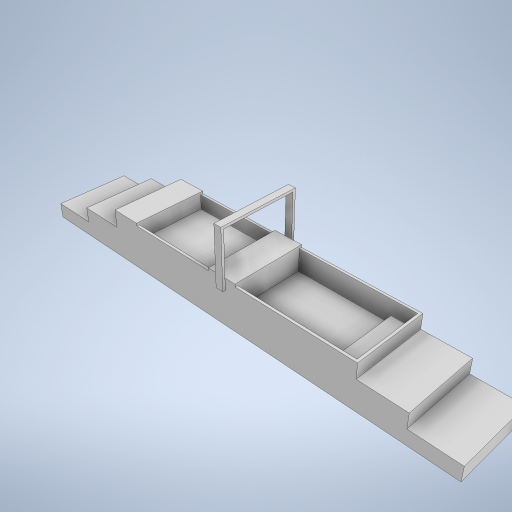
# Autodesk Inventor part: platform
Saved by Autodesk Inventor 2023 (Build 270158000, 158)
## iProperties
Created: 2022-10-30
Part Number: platform
Material: Generic
Document SubType Name: Modeling
Designer: omrfrkmll
Density: 1 g/cm^3
Appearance: Default
Author: omrfrkmll
Autodesk Inventor part; units mm, degrees
ref_plane "YZ Plane" through (0, 0, 0) normal (1, 0, 0) x (0, 1, 0)
ref_plane "XZ Plane" through (0, 0, 0) normal (0, 1, 0) x (-1, 0, 0)
ref_plane "XY Plane" through (0, 0, 0) normal (0, 0, 1) x (1, 0, 0)
sketch "Sketch1" plane through (0, 0, 0) normal (0, 0, 1) x (1, 0, 0)
  line L0 (0, 0) -> (0, 100)
  line L1 (0, 100) -> (300, 100)
  line L2 (300, 100) -> (300, 200)
  line L3 (300, 200) -> (600, 200)
  line L4 (600, 200) -> (600, 300)
  line L5 (2400, 300) -> (2400, 200)
  line L6 (2400, 200) -> (2700, 200)
  line L7 (2700, 200) -> (2700, 100)
  line L8 (2700, 100) -> (3000, 100)
  line L9 (3000, 100) -> (3000, 0)
  line L10 (3000, 0) -> (0, 0)
  line L11 (1600, 300) -> (1600, 318)
  line L12 (1600, 318) -> (1400, 318)
  line L13 (1400, 318) -> (1400, 300)
  line L14 (800, 300) -> (1400, 300)
  line L15 (1600, 300) -> (2400, 300)
  line L16 (800, 300) -> (800, 318)
  line L17 (800, 318) -> (600, 318)
  line L18 (600, 318) -> (600, 300)
  dimension "d0" = 100
  dimension "d1" = 100
  dimension "d2" = 300
  dimension "d6" = 300
  dimension "d7" = 300
  dimension "d10" = 18
  dimension "d11" = 18
  dimension "d12" = 100
  dimension "d13" = 800
  dimension "d15" = 300
  dimension "d16" = 800
  dimension "d17" = 200
  dimension "d44" = 200
  constraints: 38 end point, 14 perpendicular, 4 point on line, 2 vertical, 1 parallel
  measures "d0" distance between parallel lines of L10 L1
  measures "d1" distance between parallel lines of L1 L3
  measures "d2" distance between parallel lines of L0 L2
  measures "d6" distance between parallel lines of L5 L7
  measures "d7" distance between parallel lines of L7 L9
  measures "d10" distance between parallel lines of L12 L14
  measures "d11" distance of L11.start L11.end
  measures "d12" distance between parallel lines of L6 L15
  measures "d13" distance between parallel lines of L11 L5
  measures "d15" distance between parallel lines of L4 L2
  measures "d16" distance between parallel lines of L13 L4
  measures "d17" distance between parallel lines of L13 L11
  measures "d44" distance between parallel lines of L16 L18
extrude "Extrusion1" add sketch "Sketch1" along normal blind 500
sketch "Sketch2" plane through (1600, 300, 0) normal (0, 1, 0) x (1, 0, 0)
  line L0 (0, -18) -> (782, -18)
  line L1 (782, -18) -> (782, -482)
  line L2 (782, -482) -> (0, -482)
  line L3 (0, -482) -> (0, -18)
  line L4 (800, -500) -> (0, -500) projected
  line L5 (800, 0) -> (0, 0) projected
  line L6 (0, 0) -> (0, -500) projected
  line L7 (800, 0) -> (800, -500) projected
  point P0 (-1600, 0)
  point P1 (800, -250)
  dimension "d18" = 18
  dimension "d19" = 18
  dimension "d21" = 0
  dimension "d22" = 18
  constraints: 8 end point, 2 parallel, 1 horizontal, 1 midpoint, 1 perpendicular
  measures "d18" distance between parallel lines of L4 L2
  measures "d19" distance between parallel lines of L5 L0
  measures "d21" distance between parallel lines of L6 L3
  measures "d22" distance from line of point (800, -250) L1
extrude "Extrusion2" cut sketch "Sketch2" against normal blind 100 contours L0 L1 L2 L3
sketch "Sketch3" plane through (1600, 200, 0) normal (0, 1, 0) x (1, 0, 0)
  line L0 (0, 0) -> (0, -500) projected
  line L1 (0, -18) -> (632, -18)
  line L2 (632, -18) -> (632, -482)
  line L3 (632, -482) -> (0, -482)
  line L4 (0, -482) -> (0, -18)
  line L5 (0, -18) -> (782, -18) projected
  line L6 (782, -482) -> (0, -482) projected
  line L7 (782, -18) -> (782, -482) projected
  point P0 (-1600, 0)
  point P1 (0, -482)
  dimension "d25" = 0
  dimension "d26" = 0
  dimension "d27" = 150
  constraints: 8 end point, 2 parallel, 1 horizontal, 1 perpendicular, 1 point on line
  measures "d25" distance between parallel lines of L5 L1
  measures "d26" distance between parallel lines of L6 L3
  measures "d27" distance between parallel lines of L7 L2
extrude "Extrusion3" cut sketch "Sketch3" against normal blind 50 contours L1 L2 L3 L0
sketch "Sketch4" plane through (600, 300, 0) normal (0, 1, 0) x (1, 0, 0)
  line L0 (800, 0) -> (800, -500) projected
  line L1 (800, -18) -> (200, -18)
  line L2 (200, -18) -> (200, -482)
  line L3 (200, -482) -> (800, -482)
  line L4 (800, -482) -> (800, -18)
  line L5 (800, 0) -> (200, 0) projected
  line L6 (800, -500) -> (200, -500) projected
  line L7 (0, 0) -> (0, -500) projected
  point P0 (-600, 0)
  point P1 (800, -482)
  dimension "d30" = 18
  dimension "d31" = 18
  dimension "d32" = 200
  constraints: 8 end point, 2 parallel, 1 horizontal, 1 perpendicular, 1 point on line
  measures "d30" distance between parallel lines of L5 L1
  measures "d31" distance between parallel lines of L6 L3
  measures "d32" distance between parallel lines of L7 L2
extrude "Extrusion4" cut sketch "Sketch4" against normal blind 100
ref_plane "Work Plane1" through (1400, 238, 0) normal (0, 1, 0) x (1, 0, 0)
sketch "Sketch5" plane through (1400, 238, 0) normal (0, 1, 0) x (1, 0, 0)
  line L0 (200, 0) -> (0, 0) projected
  line L1 (125, 0) -> (75, 0)
  line L2 (75, 0) -> (75, 18)
  line L3 (75, 18) -> (125, 18)
  line L4 (125, 18) -> (125, 0)
  line L5 (0, 0) -> (0, -500) projected
  line L6 (0, -250) -> (1064.6178, -250)
  line L7 (200, -500) -> (0, -500) projected
  line L8 (100, -500) -> (100, 124.9847)
  line L9 (125, -500) -> (75, -500)
  line L10 (75, -500) -> (75, -518)
  line L11 (75, -518) -> (125, -518)
  line L12 (125, -518) -> (125, -500)
  point P0 (-1400, 0)
  dimension "d36" = 50
  dimension "d37" = 18
  constraints: 20 end point, 4 symmetric about line, 2 horizontal, 2 midpoint, 2 parallel, 1 perpendicular, 1 point on line, 1 vertical, 1 other
  measures "d36" distance between parallel lines of L4 L2
  measures "d37" distance between parallel lines of L0 L3
extrude "Extrusion5" add sketch "Sketch5" along normal blind 380 contours L2 L3 L8 L0 | L8 L3 L4 L0 | L7 L12 L11 L10
sketch "Sketch6" plane through (1475, 238, 518) normal (0, 0, 1) x (1, 0, 0)
  line L0 (0, 80) -> (0, 380) projected
  line L1 (0, 380) -> (50, 380)
  line L2 (50, 380) -> (50, 398)
  line L3 (50, 398) -> (0, 398)
  line L4 (0, 398) -> (0, 380)
  point P0 (-1475, -238)
  dimension "d40" = 18
  dimension "d41" = 50
  constraints: 8 end point, 2 parallel, 1 horizontal, 1 perpendicular
  measures "d40" distance between parallel lines of L3 L1
  measures "d41" distance between parallel lines of L2 L4
extrude "Extrusion6" add sketch "Sketch6" against normal up to surface (536 mm away)
shell "Shell1" thickness 18 removed faces 1 at (1000, 0, 166.6667)
body "Solid1"
